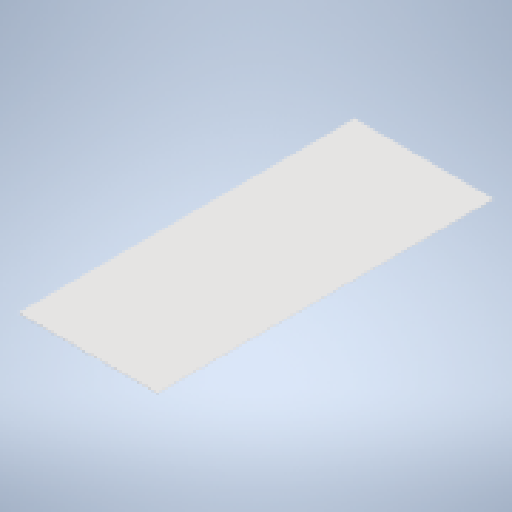
# Autodesk Inventor part: BSH 031 nose 1
Saved by Autodesk Inventor 2025 (Build 290162010, 162A)
## iProperties
Created: 2024-07-23
Part Number: BSH 031 nose 1
Material: 09g2s
Document SubType Name: Sheet Metal
Designer: admin
Density: 7.85 g/cm^3
Flat Pattern Width: 114.7 cm
Flat Pattern Length: 290 cm
Flat Pattern Area: 33263 cm^2
Sheet Metal Rule: AISI304 3mm Die 32
Sheet Metal Width: 1147,000 mm
Sheet Metal Length: 2900,000 mm
Sheet Metal Area: 3326300,000 mm^2
Appearance: Default
Author: admin
Autodesk Inventor part; units mm, degrees
ref_plane "YZ Plane" through (0, 0, 0) normal (1, 0, 0) x (0, 1, 0)
ref_plane "XZ Plane" through (0, 0, 0) normal (0, 1, 0) x (-1, 0, 0)
ref_plane "XY Plane" through (0, 0, 0) normal (0, 0, 1) x (1, 0, 0)
sketch "Sketch5" plane through (0, 0, 0) normal (0, 0, 1) x (1, 0, 0)
  line L0 (0, 2900) -> (1200, 2900)
  line L1 (1200, 2900) -> (1200, 0)
  line L2 (1200, 0) -> (0, 0)
  line L3 (0, 0) -> (0, 2900)
  line L4 (0, 2900) -> (1200, 0) construction
  line L5 (1200, 2900) -> (0, 0) construction
  line L6 (950, 0) -> (1100, 150)
  line L7 (1100, 150) -> (1147, 2900)
  point P0 (600, 1450)
  dimension "d26" = 1200
  dimension "d27" = 2900
  dimension "d29" = 53
  dimension "d30" = 950
  dimension "d31" = 150
  dimension "d32" = 100
  measures "d26" distance of L1.end L2.end
  measures "d27" distance of L0.end L1.end
  measures "d29" distance of L0.end L7.end
  measures "d30" distance of point (0, 0) L6.start
  measures "d31" distance from line of L2 L6.end
  measures "d32" distance from line of L1 L6.end
extrude "Plate4" add sketch "Sketch5" along normal blind 3 contours L0 L7 L6 L2 L3
equation "\"d28\" = Thickness"
equation "\"BendReliefWidth\" = Thickness"
equation "\"BendReliefDepth\" = 0.5 * Thickness"
equation "\"CornerReliefSize\" = 4 * Thickness"
equation "\"MinimumRemnant\" = 2 * Thickness"
equation "\"TransitionRadius\" = BendRadius"
equation "\"JacobiRadiusSize\" = BendRadius"
equation "\"GapSize\" = Thickness"
equation "\"Thickness\" = 3"
equation "\"BendRadius\" = 5"
body "Solid2"
